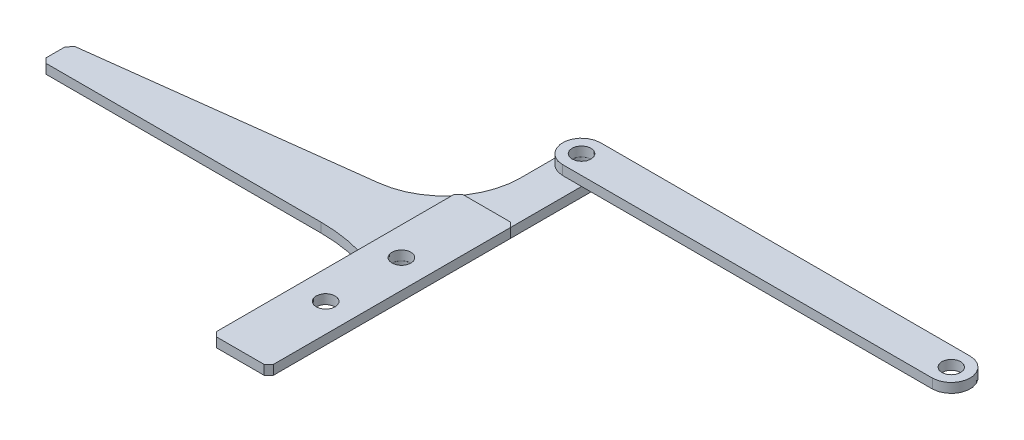
# Autodesk Inventor part: ClawPart
Saved by Autodesk Inventor 2023 (Build 270158000, 158)
## iProperties
Created: 2023-01-27
Part Number: ClawPart
Material: Generic
Document SubType Name: Modeling
Designer: Terrence
Density: 1 g/cm^3
Appearance: Default
Author: Terrence
Autodesk Inventor part; units mm, degrees
ref_plane "YZ Plane" through (0, 0, 0) normal (1, 0, 0) x (0, 1, 0)
ref_plane "XZ Plane" through (0, 0, 0) normal (0, 1, 0) x (-1, 0, 0)
ref_plane "XY Plane" through (0, 0, 0) normal (0, 0, 1) x (1, 0, 0)
sketch "Sketch1" plane through (0, 0, 0) normal (0, 1, 0) x (-1, 0, 0)
  line L0 (67.7281, -374.7602) -> (321.7281, -374.7602)
  line L1 (321.7281, -374.7602) -> (321.7281, -393.8102)
  line L2 (321.7281, -393.8102) -> (67.7281, -425.5602)
  line L3 (67.7281, -374.7602) -> (67.7281, -425.5602)
  point P0 (0, 0)
  dimension "d0" = 254
  dimension "d1" = 19.05
  dimension "d24" = 50.8
  constraints: 8 end point, 2 vertical, 1 horizontal
  measures "d0" distance of L0.start L0.end
  measures "d1" distance of L0.end L1.end
  measures "d24" distance of L0.start L2.end
extrude "Extrusion1" add sketch "Sketch1" along normal blind 6.35
sketch "Sketch3" plane through (0, 6.35, 0) normal (0, 1, 0) x (1, 0, 0)
  line L0 (-93.1281, 374.7602) -> (-67.7281, 374.7602)
  line L1 (-67.7281, 374.7602) -> (-67.7281, 508.1102)
  line L2 (-67.7281, 508.1102) -> (-93.1281, 508.1102)
  line L3 (-93.1281, 508.1102) -> (-93.1281, 374.7602)
  line L4 (-80.4281, 374.7602) -> (-80.4281, 501.7602) construction
  circle A0 centre (-80.4281, 374.7602) radius 6.35
  circle A1 centre (-80.4281, 501.7602) radius 6.35
  line L5 (-93.1281, 374.7602) -> (-67.7281, 374.7602)
  line L6 (-67.7281, 374.7602) -> (-67.7281, 362.0602)
  line L7 (-67.7281, 362.0602) -> (-93.1281, 362.0602)
  line L8 (-93.1281, 362.0602) -> (-93.1281, 374.7602)
  point P0 (0, 0)
  dimension "d25" = 127
  dimension "d26" = 12.7
  dimension "d27" = 12.7
  dimension "d28" = 133.35
  dimension "d29" = 25.4
  dimension "d30" = 25.4
  dimension "d31" = 12.7
  constraints: 18 end point, 4 parallel, 3 coincident, 2 centre point, 2 horizontal, 2 perpendicular, 1 midpoint, 1 vertical
  measures "d25" distance of L4.start L4.end
  measures "d26" diameter of A0
  measures "d27" diameter of A1
  measures "d28" distance of L0.end L1.end
  measures "d29" distance of L1.end L2.end
  measures "d30" distance of L6.end L7.end
  measures "d31" distance of L5.end L6.end
extrude "Extrusion3" add sketch "Sketch3" against normal up to surface (6.35 mm away) contours A1 | A0 L0 L3 L2 L1 | A0 L0 | L0 A0 | L0 L6 L7 L8 A0
sketch "Sketch4" plane through (0, 6.35, 0) normal (0, 1, 0) x (1, 0, 0)
  line L0 (-80.4281, 374.7602) -> (-80.4281, 495.4102) construction
  circle A0 centre (-80.4281, 374.7602) radius 6.35
  circle A1 centre (-80.4281, 495.4102) radius 6.35
  line L1 (-321.7281, 374.7602) -> (-93.1281, 374.7602) projected
  line L2 (-93.1281, 374.7602) -> (-67.7281, 374.7602) construction
  line L3 (-67.7281, 508.1102) -> (-67.7281, 362.0602) projected
  point P0 (0, 0)
  dimension "d34" = 12.7
  dimension "d35" = 12.7
  dimension "d36" = 120.65
  constraints: 4 end point, 2 centre point, 2 coincident, 1 horizontal, 1 midpoint, 1 point on line, 1 vertical
  measures "d34" diameter of A0
  measures "d35" diameter of A1
  measures "d36" distance of L0.start L0.end
extrude "Extrusion4" cut sketch "Sketch4" against normal blind 25.4
sketch "Sketch5" plane through (0, 6.35, 0) normal (0, 1, 0) x (1, 0, 0)
  line L0 (-80.4281, 323.9602) -> (-80.4281, 374.7602) construction
  circle A0 centre (-80.4281, 374.7602) radius 6.35 projected
  line L1 (-99.4781, 266.8102) -> (-99.4781, 431.9102)
  line L2 (-99.4781, 431.9102) -> (-61.3781, 431.9102)
  line L3 (-61.3781, 431.9102) -> (-61.3781, 266.8102)
  line L4 (-61.3781, 266.8102) -> (-99.4781, 266.8102)
  line L5 (-99.4781, 266.8102) -> (-61.3781, 431.9102) construction
  line L6 (-99.4781, 431.9102) -> (-61.3781, 266.8102) construction
  point P0 (0, 0)
  point P1 (-80.4281, 349.3602)
  dimension "d42" = 50.8
  dimension "d43" = 38.1
  dimension "d44" = 165.1
  constraints: 14 end point, 3 midpoint, 2 parallel, 2 vertical, 1 coincident, 1 perpendicular
  measures "d42" distance of L0.start L0.end
  measures "d43" distance of L1.end L2.end
  measures "d44" distance of L1.start L1.end
extrude "Extrusion5" add sketch "Sketch5" along normal blind 6.35 separate body contours A0 | L1 L2 L3 L4
sketch "Sketch6" plane through (0, 6.35, 0) normal (0, 1, 0) x (1, 0, 0)
  circle A0 centre (-80.4281, 495.4102) radius 6.35 projected
  circle A1 centre (-80.4281, 495.4102) radius 6.35 projected
  line L0 (-80.4281, 495.4102) -> (167.2219, 495.4102) construction
  line L1 (179.9219, 482.7102) -> (-93.1281, 482.7102)
  line L2 (-93.1281, 482.7102) -> (-93.1281, 508.1102)
  line L3 (-93.1281, 508.1102) -> (179.9219, 508.1102)
  line L4 (179.9219, 508.1102) -> (179.9219, 482.7102)
  line L5 (179.9219, 482.7102) -> (-93.1281, 508.1102) construction
  line L6 (-93.1281, 482.7102) -> (179.9219, 508.1102) construction
  circle A2 centre (167.2219, 495.4102) radius 6.35
  point P0 (0, 0)
  point P1 (43.3969, 495.4102)
  dimension "d47" = 247.65
  dimension "d48" = 273.05
  dimension "d49" = 25.4
  dimension "d55" = 12.7
  constraints: 14 end point, 3 midpoint, 3 parallel, 1 centre point, 1 coincident, 1 horizontal, 1 perpendicular
  measures "d47" distance of L0.start L0.end
  measures "d48" distance of L2.end L3.end
  measures "d49" distance of L1.end L2.end
  measures "d55" diameter of A2
extrude "Extrusion6" add sketch "Sketch6" along normal blind 6.35 separate body
ref_plane "Work Plane1" through (-99.4781, 6.35, -349.3602) normal (0, 0, 1) x (1, 0, 0)
sketch "Sketch7" plane through (0, 12.7, 0) normal (0, 1, 0) x (1, 0, 0)
  circle A0 centre (-80.4281, 374.7602) radius 6.35
  circle A1 centre (-80.4281, 374.7602) radius 6.35 projected
  point P0 (0, 0)
  dimension "d52" = 12.7
  constraints: 1 centre point, 1 coincident
  measures "d52" diameter of A0
extrude "Extrusion7" cut sketch "Sketch7" against normal blind 6.35 bodies 2
mirror "Mirror2" about plane through (-99.4781, 6.35, -349.3602) normal (0, 0, 1) of "Extrusion7" bodies 2
fillet "Fillet6" radius 50.8 1 edges at (-93.1281, 3.175, -422.3852)
fillet "Fillet6" radius 12.7 4 edges at (-93.1281, 3.175, -508.1102) (-67.7281, 3.175, -508.1102) (-93.1281, 3.175, -362.0602) (-67.7281, 3.175, -362.0602)
fillet "Fillet6" radius 107.95 1 edges at (-93.1281, 3.175, -374.7602)
chamfer "Chamfer1" distance 3.175 angle 45 2 edges at (-321.7281, 3.175, -393.8102) (-321.7281, 3.175, -374.7602)
fillet "Fillet7" radius 12.7 4 edges at (-93.1281, 9.525, -508.1102) (-93.1281, 9.525, -482.7102) (179.9219, 9.525, -508.1102) (179.9219, 9.525, -482.7102)
chamfer "Chamfer2" distance 3.175 angle 45 4 edges at (-61.3781, 9.525, -266.8102) (-61.3781, 9.525, -431.9102) (-99.4781, 9.525, -431.9102) (-99.4781, 9.525, -266.8102)
body "Solid1"
body "Solid2"
body "Solid3"
